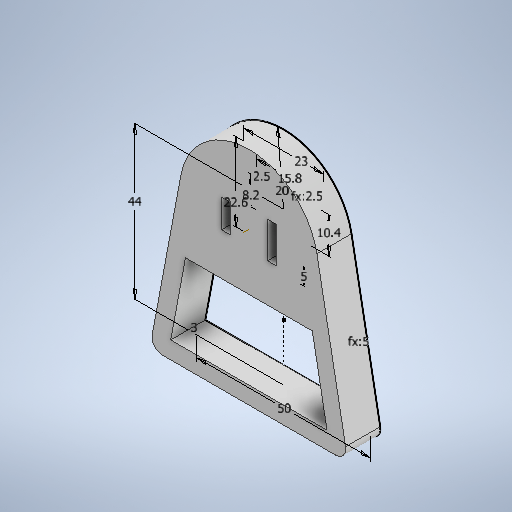
# Autodesk Inventor part: Sensor Stand
Saved by Autodesk Inventor 2026.1 (Build 301233020, 233B)
## iProperties
Created: 2025-11-03
Part Number: Sensor Stand
Material: Generic
Document SubType Name: Modeling
Designer: yo
Density: 1 g/cm^3
Appearance: Default
Author: yo
Autodesk Inventor part; units mm, degrees
ref_plane "YZ Plane" through (0, 0, 0) normal (1, 0, 0) x (0, 1, 0)
ref_plane "XZ Plane" through (0, 0, 0) normal (0, 1, 0) x (-1, 0, 0)
ref_plane "XY Plane" through (0, 0, 0) normal (0, 0, 1) x (1, 0, 0)
sketch "Sketch1" plane through (0, 0, 0) normal (0, 0, 1) x (1, 0, 0)
  line L0 (-25, 0) -> (25, 0)
  arc A0 (19.6561, 47.6928) -> (-19.6561, 47.6928) centre (0, 44) ccw
  arc A1 (-27.9484, 3.5539) -> (-25, 0) centre (-25, 3) ccw
  arc A2 (25, 0) -> (27.9484, 3.5539) centre (25, 3) ccw
  line L1 (-27.9484, 3.5539) -> (-19.6561, 47.6928)
  line L2 (19.6561, 47.6928) -> (27.9484, 3.5539)
  line L3 (-11.5, 55.3) -> (11.5, 55.3)
  line L4 (11.5, 55.3) -> (11.5, 32.7)
  line L5 (11.5, 32.7) -> (-11.5, 32.7)
  line L6 (-11.5, 32.7) -> (-11.5, 55.3)
  line L7 (-7.9, 48.1) -> (-5.4, 48.1)
  line L8 (-5.4, 48.1) -> (-5.4, 39.9)
  line L9 (-5.4, 39.9) -> (-7.9, 39.9)
  line L10 (-7.9, 39.9) -> (-7.9, 48.1)
  line L11 (5.4, 49.2) -> (7.9, 49.2)
  line L12 (7.9, 49.2) -> (7.9, 38.8)
  line L13 (7.9, 38.8) -> (5.4, 38.8)
  line L14 (5.4, 38.8) -> (5.4, 49.2)
  line L15 (-5.4, 44) -> (5.4, 44) construction
  line L16 (0, 32.7) -> (0, 0) construction
  line L17 (-18.3247, 27.7) -> (-22.5893, 5)
  line L18 (-22.5893, 5) -> (22.5893, 5)
  line L19 (22.5893, 5) -> (18.3247, 27.7)
  line L20 (18.3247, 27.7) -> (-18.3247, 27.7)
  point P0 (0, 55.3)
  point P1 (11.5, 44)
  point P2 (0, 44)
  point P3 (20.457, 16.35)
  point P4 (0, 16.35)
  point P5 (0, 27.7)
  dimension "d0" = 44
  dimension "d1" = 50
  dimension "d2" = 20
  dimension "d3" = 3
  dimension "d6" = 23
  dimension "d7" = 22.6
  dimension "d8" = 15.8
  dimension "d9" = 8.2
  dimension "d10" = 2.5
  dimension "d11" = 2.5
  dimension "d12" = 10.4
  dimension "d13" = 5
  dimension "d14" = 5
  constraints: 42 end point, 10 midpoint, 9 parallel, 6 horizontal, 6 point on circle, 6 tangent, 4 coincident, 3 centre point, 3 perpendicular, 3 vertical alignment, 2 horizontal alignment, 1 equal length, 1 vertical
  measures "d0" distance of point (0, 0) A0.centre
  measures "d1" distance of L0.start L0.end
  measures "d2" radius of A0
  measures "d3" radius of A1
  measures "d6" distance of L3.start L3.end
  measures "d7" distance of L5.end L3.start
  measures "d8" distance between parallel lines of L12 L10
  measures "d9" distance between parallel lines of L9 L7
  measures "d10" distance of L7.start L7.end
  measures "d11" distance of L11.start L11.end
  measures "d12" distance of L11.end L12.end
  measures "d13" distance between parallel lines of L5 L20
  measures "d14" distance between parallel lines of L2 L19
extrude "Extrusion1" add sketch "Sketch1" along normal blind 10 contours A1 L1 A0 L2 A2 L0 | L3 L4 L5 L6
extrude "Extrusion2" cut sketch "Sketch1" along normal blind 7.3 contours L3 L4 L5 L6
equation "\"d11\" = d10"
equation "\"d14\" = d13"
body "Solid1"
